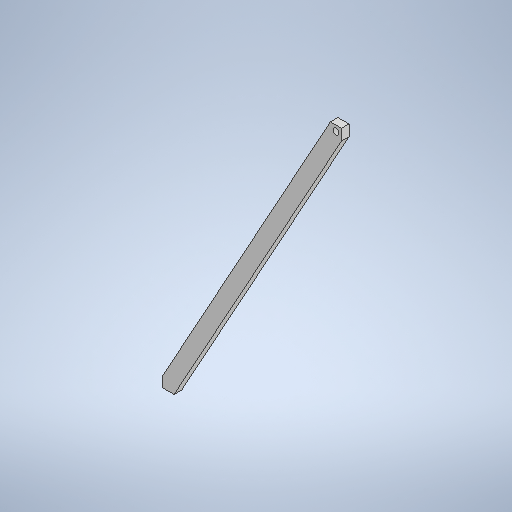
# Autodesk Inventor part: Support - Left
Saved by Autodesk Inventor 2025.2 (Build 292293000, 293)
## iProperties
Created: 2025-02-17
Part Number: Support - Left
Material: Generic
Document SubType Name: Modeling
Designer: baolo
Density: 1 g/cm^3
Appearance: Default
Author: baolo
Autodesk Inventor part; units mm, degrees
ref_plane "YZ Plane" through (0, 0, 0) normal (1, 0, 0) x (0, 1, 0)
ref_plane "XZ Plane" through (0, 0, 0) normal (0, 1, 0) x (-1, 0, 0)
ref_plane "XY Plane" through (0, 0, 0) normal (0, 0, 1) x (1, 0, 0)
sketch "Sketch1" plane through (0, 0, 0) normal (0, 0, 1) x (1, 0, 0)
  line L0 (0, 14.7186) -> (14.7186, 14.7186) construction
  line L1 (14.7186, 14.7186) -> (14.7186, 0) construction
  line L2 (14.7186, 0) -> (0, 0)
  line L3 (0, 0) -> (0, 14.7186)
  line L4 (0, 14.7186) -> (14.7186, 0) construction
  line L5 (14.7186, 14.7186) -> (0, 0) construction
  line L6 (222.3704, 417.3593) -> (237.089, 417.3593)
  line L7 (237.089, 417.3593) -> (237.089, 402.6407)
  line L8 (237.089, 402.6407) -> (222.3704, 402.6407) construction
  line L9 (222.3704, 402.6407) -> (222.3704, 417.3593) construction
  line L10 (222.3704, 417.3593) -> (237.089, 402.6407) construction
  line L11 (237.089, 417.3593) -> (222.3704, 402.6407) construction
  line L12 (222.3704, 417.3593) -> (0, 14.7186)
  line L13 (237.089, 402.6407) -> (14.7186, 0)
  line L14 (0, 0) -> (237.089, 417.3593) construction
  line L15 (-47.4178, 0) -> (284.5068, 0) construction
  point P0 (7.3593, 7.3593)
  point P1 (229.7297, 410)
  point P2 (118.5445, 208.6797)
  dimension "d1" = 480
  dimension "d14" = 410
  dimension "d15" = 20
  constraints: 30 end point, 5 midpoint, 4 parallel, 3 equal length, 2 horizontal, 2 perpendicular, 1 coincident
  measures "d1" distance of L2.end L6.end
  measures "d14" distance from line of L15 point (229.73, 410)
  measures "d15" distance between parallel lines of L13 L12
extrude "Extrusion1" add sketch "Sketch1" along normal mid plane 10
sketch "Sketch2" plane through (0, 0, 5) normal (0, 0, 1) x (1, 0, 0)
  line L0 (237.089, 417.3593) -> (222.3704, 417.3593) construction
  line L1 (237.089, 402.6407) -> (237.089, 417.3593) construction
  line L2 (222.3704, 417.3593) -> (237.089, 402.6407) construction
  point P0 (0, 0)
  point P1 (229.7297, 410)
  constraints: 2 end point, 1 midpoint
hole "Hole1" at (229.7297, 410, 5) direction (0, 0, -1) diameter 8 end through all
body "Solid1"
